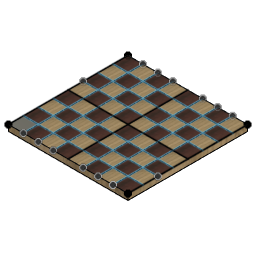
chess board v1 (Autodesk Fusion 360 design; units mm, degrees)
Autodesk Fusion 360 part; units mm, degrees
sketch "Sketch1" plane through (0, 0, 0) normal (0, 0, 1) x (1, 0, 0)
  line L0 (0, 0) -> (400, 0)
  line L1 (400, 0) -> (400, 400)
  line L2 (400, 400) -> (0, 400)
  line L3 (0, 400) -> (0, 0)
  constraint horizontal L0
  constraint vertical L1
  constraint horizontal L2
  constraint vertical L3
  constraint coincident L0.start L3.end
extrude "Extrude1" add sketch "Sketch1" along normal blind 20 makes body 1
sketch "Sketch2" plane through (0, 0, 20) normal (0, 0, 1) x (-1, 0, 0)
  line L0 (0, -400) -> (0, 0)
  line L1 (0, 0) -> (-400, 0)
  line L2 (-400, 0) -> (-400, -400)
  line L3 (-400, -400) -> (0, -400)
  line L4 (0, -400) -> (0, 0)
  line L5 (-400, 0) -> (-400, -400)
  line L6 (-50, -400) -> (-50, 0)
  line L7 (-100, -400) -> (-100, 0)
  line L8 (-150, -400) -> (-150, 0)
  line L9 (-200, 0) -> (-200, -400)
  line L10 (-250, -400) -> (-250, 0)
  line L11 (-300, 0) -> (-300, -400)
  line L12 (-350, -400) -> (-350, 0)
  line L13 (0, -50) -> (-400, -50)
  line L14 (-400, -100) -> (0, -100)
  line L15 (0, -150) -> (-400, -150)
  line L16 (-400, -200) -> (0, -200)
  line L17 (0, -250) -> (-400, -250)
  line L18 (-400, -300) -> (0, -300)
  line L19 (0, -350) -> (-400, -350)
  constraint coincident L0.start L3.end
  constraint coincident L0.end L1.start
  constraint coincident L1.end L2.start
  constraint coincident L2.end L3.start
  constraint coincident L3 L6.start
  constraint coincident L1 L6.end
  constraint perpendicular L1 L6
  constraint coincident L3 L7.start
  constraint coincident L1 L7.end
  constraint perpendicular L3 L7
  constraint coincident L3 L8.start
  constraint coincident L1 L8.end
  constraint perpendicular L1 L8
  constraint midpoint L1 L9.start
  constraint midpoint L3 L9.end
  constraint coincident L3 L10.start
  constraint coincident L1 L10.end
  constraint perpendicular L1 L10
  constraint coincident L1 L11.start
  constraint coincident L3 L11.end
  constraint perpendicular L3 L11
  constraint coincident L3 L12.start
  constraint coincident L1 L12.end
  constraint perpendicular L1 L12
  constraint coincident L4 L13.start
  constraint coincident L5 L13.end
  constraint perpendicular L5 L13
  constraint coincident L2 L14.start
  constraint coincident L4 L14.end
  constraint perpendicular L4 L14
  constraint coincident L4 L15.start
  constraint coincident L5 L15.end
  constraint perpendicular L5 L15
  constraint midpoint L5 L16.start
  constraint midpoint L4 L16.end
  constraint coincident L0 L17.start
  constraint coincident L5 L17.end
  constraint perpendicular L5 L17
  constraint coincident L5 L18.start
  constraint coincident L4 L18.end
  constraint perpendicular L4 L18
  constraint coincident L4 L19.start
  constraint coincident L5 L19.end
  constraint perpendicular L5 L19
extrude "Extrude2" add sketch "Sketch2" along normal blind 0.1 separate body contours L0 L1 L4 L6 L13 makes body 2
extrude "Extrude3" add sketch "Sketch2" along normal blind 0.1 separate body contours L0 L4 L6 L18 L19 | L3 L6 L7 L19 | L0 L4 L6 L16 L17 | L6 L7 L17 L18 | L7 L8 L18 L19 | L3 L8 L9 L19 | L0 L4 L6 L14 L15 | L6 L7 L15 L16 | L7 L8 L16 L17 | L8 L9 L17 L18 | L9 L10 L18 L19 | L3 L10 L11 L19 | L6 L7 L13 L14 | L7 L8 L14 L15 | L8 L9 L15 L16 | L9 L10 L16 L17 | L10 L11 L17 L18 | L11 L12 L18 L19 | L2 L3 L5 L12 L19 | L1 L7 L8 L13 | L8 L9 L13 L14 | L9 L10 L14 L15 | L10 L11 L15 L16 | L11 L12 L16 L17 | L2 L5 L12 L17 L18 | L1 L9 L10 L13 | L10 L11 L13 L14 | L11 L12 L14 L15 | L2 L5 L12 L15 L16 | L1 L11 L12 L13 | L2 L5 L12 L13 L14 makes body 3 at (116.6667, 33.3333, 20)
extrude "Extrude4" add sketch "Sketch2" along normal blind 0.1 separate body contours L0 L3 L4 L6 L19 | L0 L4 L6 L17 L18 | L6 L7 L18 L19 | L3 L7 L8 L19 | L0 L4 L6 L15 L16 | L6 L7 L16 L17 | L7 L8 L17 L18 | L8 L9 L18 L19 | L3 L9 L10 L19 | L0 L4 L6 L13 L14 | L6 L7 L14 L15 | L7 L8 L15 L16 | L8 L9 L16 L17 | L9 L10 L17 L18 | L10 L11 L18 L19 | L3 L11 L12 L19 | L1 L6 L7 L13 | L7 L8 L13 L14 | L8 L9 L14 L15 | L9 L10 L15 L16 | L10 L11 L16 L17 | L11 L12 L17 L18 | L2 L5 L12 L18 L19 | L1 L8 L9 L13 | L9 L10 L13 L14 | L10 L11 L14 L15 | L11 L12 L15 L16 | L2 L5 L12 L16 L17 | L1 L10 L11 L13 | L11 L12 L13 L14 | L2 L5 L12 L14 L15 | L1 L2 L5 L12 L13 makes body 4 at (66.6667, 33.3333, 20)
